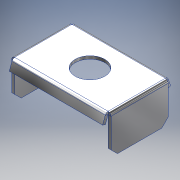
# Autodesk Inventor part: 頭_メインフレーム_1_4
Saved by Autodesk Inventor 2018 (Build 220112000, 112)
## iProperties
Created: 2016-05-11
Part Number: 頭_メインフレーム_1_4
Material: アルミニウム 5052
Document SubType Name: シート メタル
Designer: hiroaki
Density: 2.68 g/cm^3
Sheet Metal Rule: Default_mm
Appearance: アルミニウム - フラット
Mass: 7.95558 g
Surface Area: 48.454 cm^2
Volume: 2.9685 cm^3
Flat Pattern Width: 3.85131 cm
Flat Pattern Length: 8.53746 cm
Flat Pattern Area: 32.8804 cm^2
Sheet Metal Width: 38.513 mm
Sheet Metal Length: 85.375 mm
Sheet Metal Area: 3288.041 mm^2
Author: hiroaki
Autodesk Inventor part; units mm, degrees
ref_plane "YZ Plane" through (0, 0, 0) normal (1, 0, 0) x (0, 1, 0)
ref_plane "XZ Plane" through (0, 0, 0) normal (0, 1, 0) x (-1, 0, 0)
ref_plane "XY Plane" through (0, 0, 0) normal (0, 0, 1) x (1, 0, 0)
sketch "スケッチ1" plane through (0, 0, 0) normal (0, 0, 1) x (1, 0, 0)
  circle A0 centre (0, 0) radius 7.5
  line L0 (-23.65, -14.5) -> (23.65, -14.5)
  line L1 (23.65, -14.5) -> (23.65, 14.5)
  line L2 (23.65, 14.5) -> (-23.65, 14.5)
  line L3 (-23.65, 14.5) -> (-23.65, -14.5)
  line L4 (-23.65, -14.5) -> (23.65, 14.5) construction
  line L5 (23.65, -14.5) -> (-23.65, 14.5) construction
  line L6 (-19.65, 10.5) -> (-19.65, 1.5)
  line L7 (-19.65, 1.5) -> (-9.8869, 1.5)
  line L8 (-19.65, 10.5) -> (-3, 10.5)
  line L9 (-3, 10.5) -> (-3, 9.5394)
  arc A1 (-3, 9.5394) -> (-9.8869, 1.5) centre (0, 0) ccw
  line L10 (0, 0) -> (0, 14.5) construction
  line L11 (0, 0) -> (23.65, 0) construction
  line L12 (19.65, 10.5) -> (19.65, 1.5)
  line L13 (19.65, 1.5) -> (9.8869, 1.5)
  line L14 (19.65, 10.5) -> (3, 10.5)
  line L15 (3, 10.5) -> (3, 9.5394)
  arc A2 (9.8869, 1.5) -> (3, 9.5394) centre (0, 0) ccw
  line L16 (-19.65, -10.5) -> (-19.65, -1.5)
  line L17 (-19.65, -1.5) -> (-9.8869, -1.5)
  line L18 (-19.65, -10.5) -> (-3, -10.5)
  line L19 (-3, -10.5) -> (-3, -9.5394)
  arc A3 (-9.8869, -1.5) -> (-3, -9.5394) centre (0, 0) ccw
  line L20 (19.65, -10.5) -> (3, -10.5)
  arc A4 (3, -9.5394) -> (9.8869, -1.5) centre (0, 0) ccw
  line L21 (3, -10.5) -> (3, -9.5394)
  line L22 (19.65, -1.5) -> (9.8869, -1.5)
  line L23 (19.65, -10.5) -> (19.65, -1.5)
  dimension "d0" = 15
  dimension "d1" = 29
  dimension "d2" = 47.3
  dimension "d25" = 4
  dimension "d28" = 4
  dimension "d29" = 2.5
  dimension "d30" = 3
  dimension "d31" = 1.5
  constraints: 48 end point, 15 symmetric about line, 8 point on circle, 6 midpoint, 5 centre point, 2 coincident, 2 horizontal, 2 parallel, 2 perpendicular, 2 vertical, 3 other
  measures "d0" diameter of A0
  measures "d1" distance of L0.end L1.end
  measures "d2" distance of L1.end L2.end
  measures "d25" distance between parallel lines of L2 L8
  measures "d28" distance between parallel lines of L3 L6
  measures "d29" radial gap between concentric circles of A0 A1
  measures "d30" distance from line of point (0, 0) L9
  measures "d31" distance from line of L10.start L7
extrude "押し出し1" add sketch "スケッチ1" along normal blind 1.5 contours L3 L2 L1 L0 | L8 L9 A1 L7 L6 | L12 L13 A2 L15 L14 | L16 L17 A3 L19 L18 | L20 L21 A4 L22 L23
sketch "スケッチ2" plane through (23.651, -14.5, -0.001) normal (1, 0, 0) x (0, 1, 0)
  line L0 (29, 0) -> (0, 0)
  line L1 (0, 0) -> (0, -23.499)
  line L2 (0, -23.499) -> (29, -23.499)
  line L3 (29, -23.499) -> (29, 0)
  constraints: 6 end point, 1 horizontal, 1 perpendicular, 1 vertical
edge flange "フランジ1" height 25 angle 90 thickness 1.5 bend radius 0.0003 thickness toward (1, 0, 0) relief straight relief width 1.5 relief depth 0.75 edges at (23.65, 0, 0) wall of the first edge with corners at (23.651, 14.5, -0.001) (23.651, -14.5, -0.001) (23.651, -14.5, -23.5) (23.651, 14.5, -23.5)
bend "曲げ1"
corner "コーナー1"
sketch "スケッチ3" plane through (25.151, -14.5, -23.5) normal (1, 0, 0) x (0, 0, -1)
  line L0 (-23.499, 29) -> (-23.499, 0) projected
  line L1 (0, 29) -> (0, 0) projected
  line L2 (-23.499, 29) -> (0, 29) projected
  circle A0 centre (-8.5, 24.5) radius 1.55
  circle A1 centre (-8.5, 4.5) radius 1.55
  line L3 (-25, 0) -> (-25, 29) projected
  line L4 (-10.9828, 31.2255) -> (-5.5, 25.7426)
  line L5 (-5.5, 25.7426) -> (-5.5, 3.2574)
  line L6 (-5.5, 3.2574) -> (-10.9828, -2.2255)
  line L7 (-10.9828, -2.2255) -> (-10.9828, -6.9534)
  line L8 (-10.9828, -6.9534) -> (6.4787, -6.9534)
  line L9 (6.4787, -6.9534) -> (6.4787, 37.6379)
  line L10 (6.4787, 37.6379) -> (-10.9828, 37.6379)
  line L11 (-10.9828, 37.6379) -> (-10.9828, 31.2255)
  circle A2 centre (-8.5, 24.5) radius 3 construction
  line L12 (-23.5, 14.5) -> (0, 14.5) construction
  line L13 (-19.499, 25) -> (-11.5, 25)
  line L14 (-11.5, 25) -> (-11.5, 4)
  line L15 (-11.5, 4) -> (-19.499, 4)
  line L16 (-19.499, 4) -> (-19.499, 25)
  dimension "d15" = 16.5
  dimension "d16" = 3.1
  dimension "d17" = 20
  dimension "d18" = 10
  dimension "d19" = 6
  dimension "d20" = 4
  dimension "d21" = 4
  constraints: 26 end point, 6 perpendicular, 3 centre point, 3 parallel, 3 tangent, 2 symmetric about line, 1 coincident, 1 equal radius, 1 horizontal, 1 midpoint, 1 point on line, 1 vertical, 1 vertical alignment, 1 other
  measures "d15" distance from line of L3 A0.centre
  measures "d16" diameter of A0
  measures "d17" distance of A1.centre A0.centre
  measures "d18" vertical distance of L12.start A0.centre
  measures "d19" diameter of A2
  measures "d20" distance between parallel lines of L2 L13
  measures "d21" distance between parallel lines of L0 L16
extrude "押し出し2" cut sketch "スケッチ3" against normal blind 1.5 contours A0 | A1 | L11 L10 L9 L8 L7 L6 L5 L4
mirror "ミラー1" about plane through (0, 0, 0) normal (1, 0, 0) of "押し出し2", "フランジ1"
fillet "フィレット1" [suppressed]
sketch "スケッチ4" plane through (23.65, 14.5009, -0.0007) normal (0, 0.9396926, 0.3420201) x (-1, 0, 0)
  line L0 (47.3, 0) -> (0, 0)
  line L1 (0, 0) -> (0, -3.949)
  line L2 (0, -3.949) -> (47.3, -3.949)
  line L3 (47.3, -3.949) -> (47.3, 0)
  constraints: 6 end point, 1 horizontal, 1 perpendicular, 1 vertical
edge flange "フランジ2" height 5 angle 70 thickness 1.5 bend radius 0.0001 thickness toward (0, 0.9396926, 0.3420201) relief straight relief width 1.5 relief depth 0.75 corner gap 1.5 corner form 0 edges at (0, 14.5, 0) (0, -14.5, 0) wall of the first edge with corners at (-23.65, 14.5009, -0.0007) (23.65, 14.5009, -0.0007) (23.65, 15.8516, -3.7115) (-23.65, 15.8516, -3.7115)
bend "曲げ2"
corner "コーナー2"
sketch "スケッチ6" plane through (25.151, -14.5, -0.001) normal (1, 0, 0) x (0, 0, -1)
  circle A0 centre (14.999, 24.5) radius 1.55 projected
  circle A1 centre (14.999, 24.5) radius 1.55
  circle A2 centre (14.999, 4.5) radius 1.55 projected
  circle A3 centre (14.999, 4.5) radius 1.55
  point P0 (-0.001, 14.5)
  constraints: 2 centre point, 2 coincident
extrude "押し出し3" add sketch "スケッチ6" against normal up to surface (1.5 mm away)
sketch "スケッチ7" plane through (-25.151, -14.5, -0.001) normal (-1, 0, 0) x (0, 0, 1)
  circle A0 centre (-14.999, 24.5) radius 1.55 projected
  circle A1 centre (-14.999, 24.5) radius 1.55
  circle A2 centre (-14.999, 4.5) radius 1.55 projected
  circle A3 centre (-14.999, 4.5) radius 1.55
  point P0 (0.001, 14.5)
  constraints: 2 centre point, 2 coincident
extrude "押し出し4" add sketch "スケッチ7" against normal up to surface (1.5 mm away)
equation "\"d18\" = 0.5 * d17"
equation "\"d5\" = BendReliefWidth"
equation "\"d6\" = BendReliefDepth"
equation "\"d7\" = MinimumRemnant"
equation "\"d8\" = BendRadius"
equation "\"d12\" = CornerReliefSize"
equation "\"d13\" = GapSize"
equation "\"d14\" = JacobiRadiusSize"
equation "\"d44\" = Thickness"
equation "\"d33\" = BendReliefWidth"
equation "\"d34\" = BendReliefDepth"
equation "\"d35\" = MinimumRemnant"
equation "\"d36\" = BendRadius"
equation "\"d40\" = CornerReliefSize"
equation "\"d41\" = GapSize"
equation "\"d42\" = JacobiRadiusSize"
equation "\"BendRadius\" = Thickness"
equation "\"BendReliefWidth\" = Thickness"
equation "\"BendReliefDepth\" = 0.5 * Thickness"
equation "\"CornerReliefSize\" = 4 * Thickness"
equation "\"MinimumRemnant\" = 2 * Thickness"
equation "\"TransitionRadius\" = BendRadius"
equation "\"JacobiRadiusSize\" = BendRadius"
equation "\"GapSize\" = Thickness"
equation "\"Thickness\" = 1.5"
